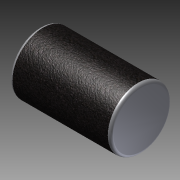
# Autodesk Inventor part: cim motor
Saved by Autodesk Inventor 2011 (Build 150239000, 239)
## iProperties
Created: 2013-01-19
Part Number: cim motor
Material: Default
Document SubType Name: Sheet Metal
Designer: Danny
Density: 1 g/cm^3
Sheet Metal Rule: Default
Author: Danny
Autodesk Inventor part; units mm, degrees
ref_plane "YZ Plane" through (0, 0, 0) normal (1, 0, 0) x (0, 1, 0)
ref_plane "XZ Plane" through (0, 0, 0) normal (0, 1, 0) x (-1, 0, 0)
ref_plane "XY Plane" through (0, 0, 0) normal (0, 0, 1) x (1, 0, 0)
sketch "Sketch1" plane through (0, 0, 0) normal (0, 0, 1) x (1, 0, 0)
  line L0 (-106.553, -66.04) -> (-3.175, -66.04)
  line L1 (0, -62.865) -> (0, -3.175)
  line L2 (-3.175, 0) -> (-106.553, 0)
  line L3 (-109.728, -3.175) -> (-109.728, -62.865)
  arc A0 (-106.553, 0) -> (-109.728, -3.175) centre (-106.553, -3.175) ccw
  arc A1 (0, -3.175) -> (-3.175, 0) centre (-3.175, -3.175) ccw
  arc A2 (-3.175, -66.04) -> (0, -62.865) centre (-3.175, -62.865) ccw
  arc A3 (-109.728, -62.865) -> (-106.553, -66.04) centre (-106.553, -62.865) ccw
  line L4 (-101.6, 0) -> (-8.128, 0)
  line L5 (-8.128, 0) -> (-8.128, -66.04)
  line L6 (-8.128, -66.04) -> (-101.6, -66.04)
  line L7 (-101.6, -66.04) -> (-101.6, 0)
  line L8 (-109.728, -33.02) -> (0, -33.02)
  line L9 (-101.6, -33.02) -> (-8.128, -33.02)
  point P0 (0, 0)
  point P1 (0, -66.04)
  point P2 (-109.728, 0)
  dimension "d0" = 109.728
  dimension "d1" = 66.04
  dimension "d2" = 3.175
  dimension "d3" = 93.472
  dimension "d4" = 66.04
  constraints: 20 end point, 8 point on circle, 8 point on line, 8 tangent, 4 centre point, 4 midpoint, 4 parallel, 3 equal radius, 2 horizontal, 2 perpendicular
  measures "d0" distance of point (-109.728, 0) point (0, 0)
  measures "d1" distance of point (0, 0) point (0, -66.04)
  measures "d2" radius of A0
  measures "d3" distance of L5.end L6.end
  measures "d4" distance of L4.end L5.end
revolve "Revolution1" add sketch "Sketch1" angle 360 about axis through (-109.728, -33.02, 0) along (1, 0, 0) contours L8 L3 A0 L2 L7 | L5 L2 A1 L1 L8
sketch "Sketch2" plane through (-101.6, -33.02, 0) normal (1, 0, 0) x (0, 0, -1)
  circle A0 centre (0, 0) radius 33.02 projected
  circle A1 centre (0, 0) radius 33.02
  point P0 (0, 33.02)
  constraints: 1 centre point, 1 coincident, 1 vertical alignment, 1 other
extrude "Extrusion1" add sketch "Sketch2" along normal blind 93.6625
sketch "Sketch3" plane through (-109.728, -33.02, 0) normal (-1, 0, 0) x (0, 0, 1)
  circle A0 centre (12.281, -11.8451) radius 1.5537
  circle A1 centre (12.281, -11.8451) radius 3.203
  circle A2 centre (18.9602, -7.3205) radius 1.5537
  circle A3 centre (18.9602, -7.3205) radius 2.8009
  point P0 (0, 33.02)
  constraints: 4 centre point, 2 coincident
extrude "Extrusion2" add sketch "Sketch3" along normal blind 1.27 contours A0
sketch "Sketch4" plane through (-109.728, -33.02, 0) normal (-1, 0, 0) x (0, 0, 1)
  circle A0 centre (17.6824, -8.7825) radius 1.5648
  point P0 (0, 33.02)
  constraints: 1 centre point
extrude "Extrusion3" add sketch "Sketch4" along normal blind 1.27
equation "\"BendRadius\" = Thickness"
equation "\"BendReliefWidth\" = Thickness"
equation "\"BendReliefDepth\" = 0.5 * Thickness"
equation "\"CornerReliefSize\" = 4 * Thickness"
equation "\"MinimumRemnant\" = 2 * Thickness"
equation "\"TransitionRadius\" = BendRadius"
equation "\"JacobiRadiusSize\" = BendRadius"
equation "\"GapSize\" = Thickness"
equation "\"Thickness\" = 3.048"
body "Solid1"
